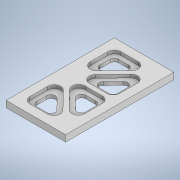
# Autodesk Inventor part: PlaskaUkrep
Saved by Autodesk Inventor 2022 (Build 260153000, 153)
## iProperties
Created: 2023-08-15
Part Number: PlaskaUkrep
Material: Generic
Document SubType Name: Modeling
Designer: Kippi
Density: 1 g/cm^3
Appearance: Default
Author: Kippi
Autodesk Inventor part; units mm, degrees
ref_plane "YZ Plane" through (0, 0, 0) normal (1, 0, 0) x (0, 1, 0)
ref_plane "XZ Plane" through (0, 0, 0) normal (0, 1, 0) x (-1, 0, 0)
ref_plane "XY Plane" through (0, 0, 0) normal (0, 0, 1) x (1, 0, 0)
sketch "Sketch1" plane through (0, 0, 0) normal (0, 1, 0) x (-1, 0, 0)
  line L0 (114.2857, 85.7143) -> (4.2857, 85.7143)
  line L1 (4.2857, 85.7143) -> (4.2857, -114.2857)
  line L2 (4.2857, -114.2857) -> (114.2857, -114.2857)
  line L3 (114.2857, -114.2857) -> (114.2857, 85.7143)
  point P0 (0, 0)
  dimension "d0" = 200
  dimension "d1" = 110
  constraints: 8 end point, 2 parallel, 1 horizontal, 1 perpendicular
  measures "d0" distance of L2.end L0.start
  measures "d1" distance of L1.end L2.end
extrude "Extrusion1" add sketch "Sketch1" along normal blind 12
sketch "Sketch2" plane through (0, 12, 0) normal (0, 1, 0) x (1, 0, 0)
  line L0 (-4.2857, -85.7143) -> (-4.2857, 114.2857) construction
  line L1 (-4.2857, 114.2857) -> (-114.2857, 114.2857) construction
  line L2 (-114.2857, 114.2857) -> (-114.2857, -85.7143) construction
  line L3 (-114.2857, -85.7143) -> (-4.2857, -85.7143) construction
  line L4 (-4.2857, -85.7143) -> (-4.2857, 114.2857) construction
  line L5 (-4.2857, 114.2857) -> (-114.2857, 114.2857) construction
  line L6 (-114.2857, 114.2857) -> (-114.2857, -85.7143) construction
  line L7 (-114.2857, -85.7143) -> (-4.2857, -85.7143) construction
  line L8 (-4.2857, -85.7143) -> (-4.2857, 114.2857) construction
  line L9 (-4.2857, 114.2857) -> (-114.2857, 114.2857) construction
  line L10 (-114.2857, 114.2857) -> (-114.2857, -85.7143) construction
  line L11 (-114.2857, -85.7143) -> (-4.2857, -85.7143) construction
  line L12 (-102.2857, -73.7143) -> (-102.2857, 102.2857)
  line L13 (-102.2857, 102.2857) -> (-16.2857, 102.2857)
  line L14 (-16.2857, 102.2857) -> (-16.2857, -73.7143)
  line L15 (-16.2857, -73.7143) -> (-102.2857, -73.7143)
  line L16 (-16.2857, -73.7143) -> (-102.2857, 14.2857)
  line L17 (-102.2857, 14.2857) -> (-16.2857, 102.2857)
  line L18 (-16.2857, 98.2857) -> (-98.2857, 98.2857)
  line L19 (-98.2857, 98.2857) -> (-98.2857, -69.7143)
  line L20 (-98.2857, -69.7143) -> (-16.2857, -69.7143)
  line L21 (-19.1465, -76.51) -> (-107.8787, 14.2857)
  line L22 (-107.8787, 14.2857) -> (-19.1465, 105.0814)
  line L23 (-20.2857, 102.2857) -> (-20.2857, -73.7143)
  line L24 (-13.425, -70.9186) -> (-96.6928, 14.2857)
  line L25 (-96.6928, 14.2857) -> (-13.425, 99.49)
  line L26 (-102.2857, 10.2857) -> (35.1189, 10.2857)
  line L27 (35.1189, 10.2857) -> (35.1189, 18.2857)
  line L28 (35.1189, 18.2857) -> (-102.2857, 18.2857)
  line L29 (-102.2857, 18.2857) -> (-102.2857, 10.2857)
  point P0 (0, 0)
  point P1 (-98.2857, 24.1017)
  point P2 (-25.7877, 98.2857)
  point P3 (-92.7837, 18.2857)
  point P4 (-20.2857, 18.2857)
  point P5 (-20.2857, 92.4697)
  point P6 (-20.2857, 10.2857)
  point P7 (-92.7837, 10.2857)
  point P8 (-20.2857, -63.8983)
  point P9 (-25.7877, -69.7143)
  point P10 (-98.2857, 4.4697)
  dimension "d4" = 12
  dimension "d5" = 4
  dimension "d6" = 4
  dimension "d7" = 4
  dimension "d8" = 4
  dimension "d9" = 4
  dimension "d10" = 4
  constraints: 36 end point, 3 parallel, 1 horizontal, 1 midpoint, 1 perpendicular, 1 point on line, 7 other
  measures "d4" distance between parallel lines of L2 L12
  measures "d5" distance between parallel lines of L12 L19
  measures "d6" distance between parallel lines of L16 L21
  measures "d7" distance between parallel lines of L14 L23
  measures "d8" distance between parallel lines of L24 L16
  measures "d9" distance from line of L28 L16.end
  measures "d10" distance from line of L26 L16.end
extrude "Extrusion2" cut sketch "Sketch2" against normal blind 6 contours L21 L20 L19 | L26 L23 L24 | L19 L18 L22 | L25 L23 L28
sketch "Sketch3" plane through (0, 6, 0) normal (0, 1, 0) x (1, 0, 0)
  line L0 (-98.2857, -69.7143) -> (-98.2857, 4.4697) construction
  line L1 (-25.7877, -69.7143) -> (-98.2857, -69.7143) projected
  line L2 (-98.2857, 4.4697) -> (-25.7877, -69.7143) construction
  line L3 (-98.2857, -69.7143) -> (-98.2857, 4.4697) construction
  line L4 (-25.7877, -69.7143) -> (-98.2857, -69.7143) construction
  line L5 (-98.2857, 4.4697) -> (-25.7877, -69.7143) construction
  line L6 (-20.2857, -63.8983) -> (-92.7837, 10.2857) construction
  line L7 (-20.2857, 10.2857) -> (-20.2857, -63.8983) construction
  line L8 (-92.7837, 10.2857) -> (-20.2857, 10.2857) construction
  line L9 (-20.2857, 92.4697) -> (-20.2857, 18.2857) construction
  line L10 (-92.7837, 18.2857) -> (-20.2857, 92.4697) construction
  line L11 (-20.2857, 18.2857) -> (-92.7837, 18.2857) construction
  line L12 (-98.2857, 98.2857) -> (-25.7877, 98.2857) construction
  line L13 (-98.2857, 24.1017) -> (-98.2857, 98.2857) construction
  line L14 (-25.7877, 98.2857) -> (-98.2857, 24.1017) construction
  line L15 (-90.2857, -15.1624) -> (-90.2857, -61.7143)
  line L16 (-90.2857, -61.7143) -> (-44.7918, -61.7143)
  line L17 (-44.7918, -61.7143) -> (-90.2857, -15.1624)
  line L18 (-73.7796, 2.2857) -> (-28.2857, -44.2662)
  line L19 (-28.2857, -44.2662) -> (-28.2857, 2.2857)
  line L20 (-28.2857, 2.2857) -> (-73.7796, 2.2857)
  line L21 (-28.2857, 72.8376) -> (-28.2857, 26.2857)
  line L22 (-28.2857, 26.2857) -> (-73.7796, 26.2857)
  line L23 (-73.7796, 26.2857) -> (-28.2857, 72.8376)
  line L24 (-90.2857, 90.2857) -> (-44.7918, 90.2857)
  line L25 (-44.7918, 90.2857) -> (-90.2857, 43.7338)
  line L26 (-90.2857, 43.7338) -> (-90.2857, 90.2857)
  point P0 (0, 0)
  dimension "d13" = 8
  dimension "d14" = 8
  dimension "d15" = 8
  dimension "d16" = 8
  constraints: 24 end point, 8 other
  measures "d13" distance between parallel lines of L13 L26
  measures "d14" distance between parallel lines of L10 L23
  measures "d15" distance between parallel lines of L8 L20
  measures "d16" distance between parallel lines of L0 L15
extrude "Extrusion3" cut sketch "Sketch3" against normal blind 6
fillet "Fillet1" radius 8 12 edges at (-90.2857, 3, -90.2857) (-73.7796, 3, -2.2857) (-73.7796, 3, -26.2857) (-90.2857, 3, 61.7143) (-90.2857, 3, -43.7338) (-44.7918, 3, 61.7143) (-28.2857, 3, 44.2662) (-28.2857, 3, -2.2857) (-90.2857, 3, 15.1624) (-28.2857, 3, -26.2857) (-28.2857, 3, -72.8376) (-44.7918, 3, -90.2857)
fillet "Fillet2" radius 12 12 edges at (-98.2857, 9, -24.1017) (-98.2857, 9, 69.7143) (-25.7877, 9, 69.7143) (-20.2857, 9, 63.8983) (-20.2857, 9, -10.2857) (-20.2857, 9, -92.4697) (-20.2857, 9, -18.2857) (-92.7837, 9, -10.2857) (-92.7837, 9, -18.2857) (-98.2857, 9, -4.4697) (-98.2857, 9, -98.2857) (-25.7877, 9, -98.2857)
body "Solid1"
